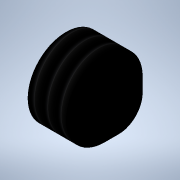
# Autodesk Inventor part: Hexagon socket set screw with flat point DIN 913 - M4x3
Saved by Autodesk Inventor 2021 (Build 250183000, 183)
## iProperties
Created: 2025-04-04
Part Number: Hexagon socket set screw with flat point DIN 913 - M4x3
Material: Generic
Catalog Web Link: www.cadenas.de
Description: DIN 913-Hexagon socket set screw with flat point
Vendor: MISUMI
Document SubType Name: Modeling
Designer: psAdmin
Manufacturer: MISUMI
Mass: 0.0287636 g
Surface Area: 0.64306 cm^2
Volume: 0.0287636 cm^3
Density: 1 g/cm^3
Appearance: PSOLRGB-0-0-0
Category: PARTsolutions
Company: MISUMI
Title: Hexagon socket set screw with flat point DIN 913 - M4x3
Author: Cadenas PARTsolutions
Comments: Hexagon socket set screw with flat point
PSOL_IDENT_0: {$CADENAS_DATA/23d-libs/misumi/metric/accessories/din_913.prj},252 {VTYP=3D},{NB=Hexagon socket set
PSOL_IDENT_1: screw with flat point DIN 913 - M4x3},{LINA=Hexagon socket set screw with flat point DIN 913 - M4x3}
PSOL_IDENT_2: ,{NN=DIN 913},{DATE=29.11.2024 04:47:06},{GEOMDATE=17.02.2014 00:00:00},{VERSION=},{LINEID=320},{WBV
PSOL_IDENT_3: AR=},{WBNUMERIC=}  {NB=Gewindestift DIN 913 - M4x3},{LINA=Gewindestift DIN 913 - M4x3},{KT=X},{IDNR=
PSOL_IDENT_4: },{NENN=M4x3},{D=4.000},{D3=3.141},{P=0.700},{L=3.000},{DP=2.500},{S=2.000},{T=1.500}
NB: Headless pin DIN 913 - M4x3
NN: DIN 913
NT: Hexagon socket set screw with flat point
NBSYN: Headless pin DIN 913 - $NENN.
LINA: Headless pin DIN 913 - M4x3
CATALOG: Misumi
ROWDESC: M4x3
D: 4
D3: 3.141
P: 0.7
L: 3
DP: 2.5
S: 2
T: 1.5
SUPPLIER: MISUMI
ARTICLENO: Hexagon socket set screw with flat point DIN 913 - M4x3
BOMINFO: Hexagon socket set screw with flat point DIN 913 - M4x3
CREATOR: CADENAS GmbH
Autodesk Inventor part; units mm, degrees
sketch "Sketch_1" plane through (0, 0, 0) normal (0, 0, 1) x (1, 0, 0)
  line L0 (0.6667, 0) -> (3, 0)
  line L1 (3, 0) -> (3, -1.25)
  line L2 (3, -1.25) -> (2.25, -2)
  line L3 (2.25, -2) -> (0.248, -2)
  line L4 (0.248, -2) -> (0, -1.5705)
  line L5 (0, -1.5705) -> (0, -1.1547)
  line L6 (0, -1.1547) -> (0.6667, 0)
  line L7 (0.6667, 0) -> (3, 0)
  constraints: 16 end point
revolve "Revolution1" add sketch "Sketch_1" angle 360 about axis through (0.6667, 0, 0) along (1, 0, 0)
thread "Thread1" size "M4x0.7" class "6g" standard "ISO Metric profile" full length
sketch "Sketch_2" plane through (0, 0, 0) normal (1, 0, 0) x (0, 1, 0)
  line L0 (0, 1.1547) -> (-1, 0.5774)
  line L1 (-1, 0.5774) -> (-1, -0.5774)
  line L2 (-1, -0.5774) -> (0, -1.1547)
  line L3 (0, -1.1547) -> (1, -0.5774)
  line L4 (1, -0.5774) -> (1, 0.5774)
  line L5 (1, 0.5774) -> (0, 1.1547)
  constraints: 12 end point
extrude "Extrusion1" cut sketch "Sketch_2" along normal blind 1.5
ref_plane "IP1_XY" through (0, 0, 0) normal (1, 0, 0) x (0, 0, -1)
ref_plane "IP1_YZ" through (0, 0, 0) normal (0, 0, -1) x (0, 1, 0)
ref_plane "IP1_ZX" through (0, 0, 0) normal (0, 1, 0) x (1, 0, 0)
ref_plane "IP2_XY" through (3, 0, 0) normal (1, 0, 0) x (0, 0, -1)
ref_plane "IP2_YZ" through (3, 0, 0) normal (0, 0, -1) x (0, 1, 0)
ref_plane "IP2_ZX" through (3, 0, 0) normal (0, 1, 0) x (1, 0, 0)
body "Solid1"
